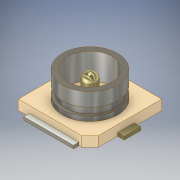
# Autodesk Inventor part: U.FL_Male
Saved by Autodesk Inventor 2017 (Build 210142000, 142)
## iProperties
Created: 2016-08-03
Part Number: U.FL_Male
Material: ABS Plastic
Document SubType Name: Modeling
Designer: Bradley
Density: 1.06 g/cm^3
Appearance: Smooth - Off-White
Description: SD-73412-011
Author: Bradley
Autodesk Inventor part; units mm, degrees
ref_plane "YZ Plane" through (0, 0, 0) normal (1, 0, 0) x (0, 1, 0)
ref_plane "XZ Plane" through (0, 0, 0) normal (0, 1, 0) x (-1, 0, 0)
ref_plane "XY Plane" through (0, 0, 0) normal (0, 0, 1) x (1, 0, 0)
sketch "Sketch1" plane through (0, 0, 0) normal (0, 0, 1) x (1, 0, 0)
  line L0 (0, 0.615) -> (0, -0.615)
  arc A0 (0.25, 0.365) -> (0, 0.615) centre (0, 0.365) ccw
  line L1 (0.25, 0.365) -> (0.25, -0.255)
  line L2 (0.25, -0.255) -> (0.8, -0.255)
  line L3 (0.8, -0.255) -> (0.8, 0.685)
  line L4 (0.8, 0.685) -> (1, 0.685)
  line L5 (1, 0.685) -> (1, 0.195)
  line L6 (1, 0.195) -> (0.9, 0.195)
  line L7 (0.9, 0.195) -> (0.9, -0.085)
  line L8 (0.9, -0.085) -> (1, -0.085)
  line L9 (1, -0.085) -> (1, -0.615)
  line L10 (1, -0.615) -> (0, -0.615)
  point P0 (0, 0)
  point P1 (0, 0)
  dimension "d0" = 1.23
  dimension "d1" = 0.5
  dimension "d2" = 1.6
  dimension "d3" = 2
  dimension "d4" = 1.3
  dimension "d5" = 0.49
  dimension "d6" = 0.28
  dimension "d7" = 0.1
  dimension "d8" = 0.36
  constraints: 22 end point, 8 perpendicular, 3 point on line, 2 point on circle, 2 vertical, 1 centre point, 1 coincident, 1 midpoint, 1 tangent
  measures "d0" distance of L0.start L0.end
  measures "d1" diameter of L1 L0
  measures "d2" diameter of L3 L0
  measures "d3" diameter of L5 L0
  measures "d4" distance between parallel lines of L10 L4
  measures "d5" distance of L4.end L5.end
  measures "d6" distance of L6.end L7.end
  measures "d7" distance between parallel lines of L5 L7
  measures "d8" distance between parallel lines of L10 L2
revolve "Revolution1" add sketch "Sketch1" angle 360 about axis through (0, 0.615, 0) along (0, -1, 0)
sketch "Sketch2" plane through (0, -0.615, 0) normal (0, -1, 0) x (1, 0, 0)
  line L0 (-1.3, -1.3) -> (1.3, -1.3)
  line L1 (1.3, -1.3) -> (1.3, 1)
  line L2 (1, 1.3) -> (-1.3, 1.3)
  line L3 (-1.3, 1.3) -> (-1.3, -1.3)
  circle A0 centre (0, 0) radius 0.25 projected
  line L4 (-1.3, -1.3) -> (1.3, 1.3) construction
  line L5 (1.3, -1.3) -> (-1.3, 1.3) construction
  line L6 (1, 1.3) -> (1.3, 1)
  point P0 (0, 0)
  dimension "d10" = 2.6
  dimension "d11" = 0.3
  dimension "d12" = 0.3
  constraints: 14 end point, 2 midpoint, 2 parallel, 2 perpendicular, 2 point on line, 1 horizontal
  measures "d10" distance of L2.end L4.end
  measures "d11" distance of L2.start L4.end
  measures "d12" distance of L1.end L4.end
extrude "Extrusion1" add sketch "Sketch2" against normal blind 0.36 contours L3 L2 L6 L1 L0 | A0
sketch "Sketch3" plane through (-1.3, -0.615, -1.3) normal (0, -1, 0) x (1, 0, 0)
  line L0 (0, 0) -> (2.6, 0) projected
  line L1 (2.6, 0) -> (2.6, 2.3) projected
  line L2 (2.6, 2.3) -> (2.3, 2.6) projected
  line L3 (2.3, 2.6) -> (0, 2.6) projected
  line L4 (0, 2.6) -> (0, 0) projected
  line L5 (2.84, 1.6) -> (2.84, 1)
  line L6 (2.84, 1) -> (1.8, 1)
  line L7 (1.8, 1) -> (1.7, 0.9)
  line L8 (1.7, 0.9) -> (0.9, 0.9)
  line L9 (0.9, 0.9) -> (0.8, 1)
  line L10 (0.8, 1) -> (0.8, 1.6)
  line L11 (0.8, 1.6) -> (0.9, 1.7)
  line L12 (0.9, 1.7) -> (1.7, 1.7)
  line L13 (1.7, 1.7) -> (1.8, 1.6)
  line L14 (1.8, 1.6) -> (2.84, 1.6)
  line L15 (-0.24, 1) -> (0.49, 1)
  line L16 (-0.24, 1) -> (-0.24, 1.6)
  line L17 (-0.24, 1.6) -> (0.49, 1.6)
  line L18 (1.525, 2.134) -> (1.525, 2.45)
  line L19 (1.525, 2.45) -> (2.2, 2.45)
  line L20 (2.2, 2.45) -> (2.2, 2.8)
  line L21 (2.2, 2.8) -> (0.4, 2.8)
  line L22 (0.4, 2.8) -> (0.4, 2.45)
  line L23 (0.4, 2.45) -> (1.075, 2.45)
  line L24 (1.075, 2.45) -> (1.075, 2.134)
  line L25 (1.525, 0.466) -> (1.525, 0.15)
  line L26 (1.525, 0.15) -> (2.2, 0.15)
  line L27 (2.2, 0.15) -> (2.2, -0.2)
  line L28 (2.2, -0.2) -> (0.4, -0.2)
  line L29 (0.4, -0.2) -> (0.4, 0.15)
  line L30 (0.4, 0.15) -> (1.075, 0.15)
  line L31 (1.075, 0.15) -> (1.075, 0.466)
  arc A0 (1.525, 2.134) -> (1.075, 2.134) centre (1.3, 1.3) ccw
  arc A1 (0.49, 1.6) -> (0.49, 1) centre (1.3, 1.3) ccw
  arc A2 (1.075, 0.466) -> (1.525, 0.466) centre (1.3, 1.3) ccw
  line L32 (1.3, 0) -> (1.3, 2.6) construction
  line L33 (0, 2.6) -> (2.3, 2.6) construction
  point P0 (1.3, 1.7)
  point P1 (1.3, 0.9)
  point P2 (1.3, -0.2)
  point P3 (1.3, 2.8)
  point P4 (0.8, 1.3)
  point P5 (2.84, 1.3)
  point P6 (-0.24, 1.3)
  dimension "d15" = 3
  dimension "d16" = 0.35
  dimension "d17" = 1.8
  dimension "d18" = 0.45
  dimension "d19" = 0.6
  dimension "d20" = 3.08
  dimension "d21" = 0.73
  dimension "d22" = 0.8
  dimension "d23" = 1
  constraints: 56 end point, 16 perpendicular, 11 equal length, 8 midpoint, 6 point on circle, 4 point on line, 4 vertical, 4 vertical alignment, 3 centre point, 3 coincident, 3 horizontal alignment, 3 parallel, 2 concentric, 2 horizontal, 1 collinear, 1 other
  measures "d15" distance between parallel lines of L21 L28
  measures "d16" distance of L21.end L22.end
  measures "d17" distance of L20.end L21.end
  measures "d18" distance between parallel lines of L24 L18
  measures "d19" distance of L5.start L5.end
  measures "d20" distance between parallel lines of L16 L5
  measures "d21" distance of L15.start L15.end
  measures "d22" distance between parallel lines of L8 L12
  measures "d23" distance from line of L10 L6.end
extrude "Extrusion2" add sketch "Sketch3" along normal blind 0.01 and the other way blind 0.11 contours L29 L30 L31 A2 L25 L26 L27 L0 | L0 L27 L28 L29 | L15 L16 L17 L4 | L4 L17 A1 L15 | L6 L7 L8 L9 L10 L11 L12 L13 L14 L1 | L1 L14 L5 L6 | L22 L21 L20 L3 | L3 L20 L19 L18 A0 L24 L23 L22
equation "\"d12\" = d11"
body "Solid1"
